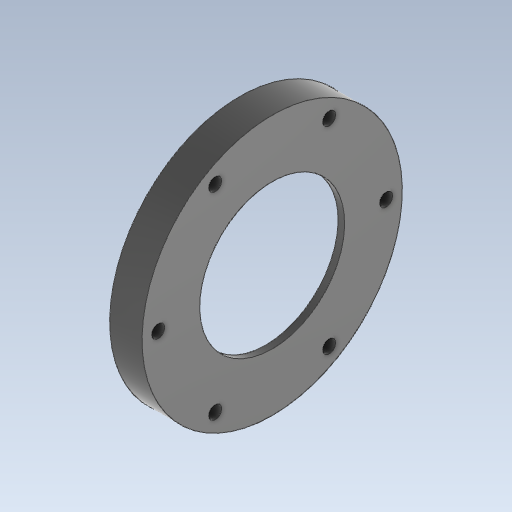
# Autodesk Inventor part: Hand_
Saved by Autodesk Inventor 2020.4 (Build 244396000, 396)
## iProperties
Created: 2022-01-10
Part Number: Hand_
Material: PC/ABS プラスチック
Document SubType Name: Modeling
Designer: Masato Kubotera
Density: 0.357273 g/cm^3
Appearance: 滑らか - 黒
Author: Masato Kubotera
Autodesk Inventor part; units mm, degrees
ref_plane "YZ Plane" through (0, 0, 0) normal (1, 0, 0) x (0, 1, 0)
ref_plane "XZ Plane" through (0, 0, 0) normal (0, 1, 0) x (-1, 0, 0)
ref_plane "XY Plane" through (0, 0, 0) normal (0, 0, 1) x (1, 0, 0)
derived "ForeArm_outside_frame_.ipt"
sketch "スケッチ1" plane through (0, 0, 0) normal (0, 1, 0) x (-1, 0, 0)
  circle A0 centre (0, 0) radius 5.05
  line L0 (0, 8.5) -> (0, -8.5) construction
  circle A1 centre (0, 8.5) radius 1.35
  circle A2 centre (-8.5, 0) radius 1.35
  circle A3 centre (0, -8.5) radius 1.35
  circle A4 centre (8.5, 0) radius 1.35
  circle A5 centre (0, -158.8519) radius 16
  line L1 (0, 0) -> (0, -158.8519) construction
  arc A6 (-16, -121.8654) -> (16, -121.8654) centre (0, -158.8519) ccw
  circle A7 centre (0, 8.5) radius 2.4 construction
  line L2 (-16, 31) -> (16, 31) construction
  line L3 (16, 31) -> (16, -12) construction
  line L4 (16, -12) -> (-16, -12) construction
  line L5 (-16, -12) -> (-16, 31) construction
  line L6 (-16, 31) -> (16, -12) construction
  line L7 (16, 31) -> (-16, -12) construction
  arc A8 (-16, 0) -> (-10.583, -12) centre (0, 0) ccw construction
  arc A9 (10.583, -12) -> (16, 0) centre (0, 0) ccw construction
  line L8 (-16, -121.8654) -> (-16, 0)
  line L9 (16, -121.8654) -> (16, 0)
  circle A10 centre (0, -92.5) radius 1.6
  line L10 (0, -158.8519) -> (-20.1494, -123.952) construction
  circle A11 centre (-17.6494, -128.2822) radius 5 construction
  circle A12 centre (-17.6494, -128.2822) radius 2
  circle A13 centre (-35.2989, -158.8519) radius 2
  circle A14 centre (-17.6494, -189.4216) radius 2
  circle A15 centre (17.6494, -189.4216) radius 2
  circle A16 centre (35.2989, -158.8519) radius 2
  circle A17 centre (17.6494, -128.2822) radius 2
  circle A18 centre (0, -158.8519) radius 58.8961 construction
  line L11 (30.6064, -21.0119) -> (2.8936, -37.0119) construction
  line L12 (2.8936, -37.0119) -> (-18.6064, 0.2272) construction
  line L13 (-18.6064, 0.2272) -> (9.1064, 16.2272) construction
  line L14 (9.1064, 16.2272) -> (30.6064, -21.0119) construction
  line L15 (30.6064, -21.0119) -> (-18.6064, 0.2272) construction
  line L16 (2.8936, -37.0119) -> (9.1064, 16.2272) construction
  line L17 (16.75, -29.0119) -> (-4.75, 8.2272) construction
  circle A19 centre (0, -42.5) radius 1.6
  line L18 (-2.5, -47.5) -> (2.5, -47.5) construction
  line L19 (2.5, -47.5) -> (2.5, -57.5) construction
  line L20 (2.5, -57.5) -> (-2.5, -57.5) construction
  line L21 (-2.5, -57.5) -> (-2.5, -47.5) construction
  line L22 (-2.5, -47.5) -> (2.5, -57.5) construction
  line L23 (2.5, -47.5) -> (-2.5, -57.5) construction
  line L24 (-2.5, -52.5) -> (2.5, -52.5) construction
  circle A20 centre (0, -62.5) radius 1.6
  line L25 (2.8936, -37.0119) -> (54.9285, -127.1389) construction
  line L26 (0, -158.8519) -> (54.9285, -127.1389) construction
  line L27 (-2.5, -47.5) -> (2.5, -47.5) construction
  line L28 (2.5, -47.5) -> (2.5, -87.5) construction
  line L29 (2.5, -87.5) -> (-2.5, -87.5) construction
  line L30 (-2.5, -87.5) -> (-2.5, -47.5) construction
  line L31 (-2.5, -47.5) -> (2.5, -87.5) construction
  line L32 (2.5, -47.5) -> (-2.5, -87.5) construction
  line L33 (-2.55, -47.45) -> (2.55, -47.45)
  line L34 (2.55, -47.45) -> (2.55, -87.55)
  line L35 (2.55, -87.55) -> (-2.55, -87.55)
  line L36 (-2.55, -87.55) -> (-2.55, -47.45)
  line L37 (-2.55, -47.45) -> (2.55, -87.55) construction
  line L38 (2.55, -47.45) -> (-2.55, -87.55) construction
  arc A21 (-1.0651, -47.45) -> (-2.55, -48.9349) centre (-1.8075, -48.1925) ccw
  arc A22 (2.55, -48.9349) -> (1.0651, -47.45) centre (1.8075, -48.1925) ccw
  line L39 (-2.5, -67.5) -> (2.5, -67.5) construction
  arc A23 (-2.55, -86.0651) -> (-1.0651, -87.55) centre (-1.8075, -86.8075) ccw
  arc A24 (1.0651, -87.55) -> (2.55, -86.0651) centre (1.8075, -86.8075) ccw
  arc A25 (16, 0) -> (-16, 0) centre (0, 0) ccw
  circle A26 centre (0, -158.8519) radius 30.2989
  point P0 (0, 9.5)
  point P1 (0, 9.5)
  point P2 (6, -10.3923)
  point P3 (0, -52.5)
  point P4 (0, -67.5)
  point P5 (0, -199.1508)
sketch "スケッチ2" plane through (0, 0, 0) normal (1, 0, 0) x (0, 1, 0)
  line L0 (0, -158.8519) -> (-63, -158.8519)
  circle A0 centre (-63, -158.8519) radius 65
  line L1 (0, -199.1508) -> (0, -121.8654) projected
  line L2 (0, -199.1508) -> (-12, -199.1508)
  line L3 (-10, -158.8519) -> (-10, -199.1508)
  line L4 (-2, -181.3018) -> (0, -181.3018)
  point P0 (0, 0)
  point P1 (-12, -158.8519)
  point P2 (-15, -202.6811)
  point P3 (0, -174.8519)
  point P4 (-10, -196.4817)
  dimension "d1" = 63
  dimension "d2" = 130
  dimension "d8" = 2
  dimension "d11" = 2
  constraints: 9 end point, 5 point on line, 3 point on circle, 2 horizontal, 2 perpendicular, 1 centre point, 1 coincident
  measures "d1" distance of L0.start L0.end
  measures "d2" diameter of A0
  measures "d8" distance of L2.end L3.end
  measures "d11" distance of L4.start L4.end
revolve "回転1" add sketch "スケッチ2" angle 360 about axis through (0, 0, -158.8519) along (0, -1, 0) contours A0 L4 L1 L2 L3
extrude "押し出し1" cut sketch "スケッチ1" against normal blind 5 contours A12 | A13 | A14 | A15 | A16 | A17
equation "\"d11\" = d8"
